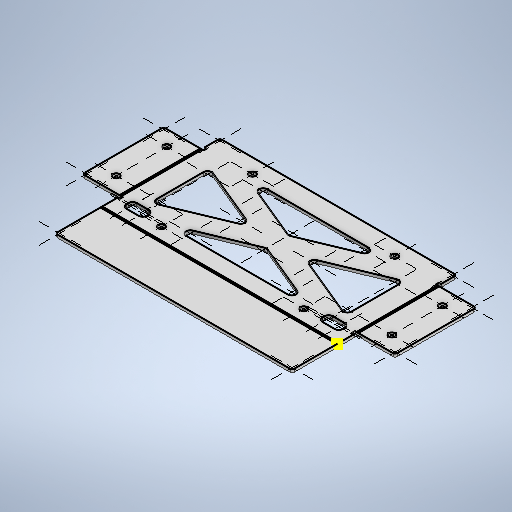
# Autodesk Inventor part: body_back_frame
Saved by Autodesk Inventor 2026.1 (Build 301233000, 233)
## iProperties
Created: 2025-08-15
Part Number: body_back_frame
Material: Generic
Document SubType Name: Modeling
Designer: chris
Density: 1 g/cm^3
Appearance: Default
Author: chris
Autodesk Inventor part; units mm, degrees
ref_plane "YZ Plane" through (0, 0, 0) normal (1, 0, 0) x (0, 1, 0)
ref_plane "XZ Plane" through (0, 0, 0) normal (0, 1, 0) x (-1, 0, 0)
ref_plane "XY Plane" through (0, 0, 0) normal (0, 0, 1) x (1, 0, 0)
sketch "Sketch1" plane through (0, 0, 0) normal (0, 1, 0) x (-1, 0, 0)
  line L0 (117, -0.4496) -> (0, -0.4496)
  line L1 (-0.1396, -9.9943) -> (-0.1396, -49.9943)
  line L2 (117.1396, -49.9943) -> (117.1396, -9.9943)
  circle A0 centre (93.69, -51.8993) radius 1.55
  circle A1 centre (23.31, -51.8993) radius 1.55
  circle A2 centre (93.69, -6.8993) radius 1.55
  circle A3 centre (23.31, -6.8993) radius 1.55
  arc A4 (15, -7.8993) -> (13, -5.8993) centre (13, -7.8993) ccw
  line L3 (7, -5.8993) -> (13, -5.8993)
  arc A5 (13, -10.8993) -> (15, -8.8993) centre (13, -8.8993) ccw
  line L4 (15, -7.8993) -> (15, -8.8993)
  arc A6 (5, -8.8993) -> (7, -10.8993) centre (7, -8.8993) ccw
  line L5 (5, -8.8993) -> (5, -7.8993)
  arc A7 (7, -5.8993) -> (5, -7.8993) centre (7, -7.8993) ccw
  arc A8 (110, -10.8993) -> (112, -8.8993) centre (110, -8.8993) ccw
  line L6 (112, -7.8993) -> (112, -8.8993)
  arc A9 (102, -8.8993) -> (104, -10.8993) centre (104, -8.8993) ccw
  line L7 (102, -8.8993) -> (102, -7.8993)
  arc A10 (112, -7.8993) -> (110, -5.8993) centre (110, -7.8993) ccw
  line L8 (104, -5.8993) -> (110, -5.8993)
  arc A11 (104, -5.8993) -> (102, -7.8993) centre (104, -7.8993) ccw
  arc A12 (13.0766, -15.651) -> (10.31, -17.4982) centre (12.31, -17.4982) ccw
  line L9 (10.31, -40.6803) -> (10.31, -17.4982)
  arc A13 (41.0052, -30.9365) -> (41.0052, -27.2421) centre (40.2386, -29.0893) ccw
  line L10 (13.0766, -15.651) -> (41.0052, -27.2421)
  arc A14 (10.31, -40.6803) -> (13.0766, -42.5275) centre (12.31, -40.6803) ccw
  line L11 (41.0052, -30.9365) -> (13.0766, -42.5275)
  arc A15 (32.6238, -45.2421) -> (33.3904, -49.0893) centre (33.3904, -47.0893) ccw
  line L12 (32.6238, -45.2421) -> (57.7334, -34.821)
  arc A16 (83.6096, -49.0893) -> (84.3762, -45.2421) centre (83.6096, -47.0893) ccw
  line L13 (59.2666, -34.821) -> (84.3762, -45.2421)
  arc A17 (59.2666, -34.821) -> (57.7334, -34.821) centre (58.5, -36.6682) ccw
  arc A18 (75.9948, -27.2421) -> (75.9948, -30.9365) centre (76.7614, -29.0893) ccw
  line L14 (75.9948, -27.2421) -> (103.9234, -15.651)
  arc A19 (106.69, -17.4982) -> (103.9234, -15.651) centre (104.69, -17.4982) ccw
  line L15 (106.69, -17.4982) -> (106.69, -40.6803)
  arc A20 (103.9234, -42.5275) -> (106.69, -40.6803) centre (104.69, -40.6803) ccw
  arc A21 (57.7334, -23.3576) -> (59.2666, -23.3576) centre (58.5, -21.5104) ccw
  line L16 (84.3762, -12.9365) -> (59.2666, -23.3576)
  arc A22 (84.3762, -12.9365) -> (83.6096, -9.0893) centre (83.6096, -11.0893) ccw
  line L17 (33.3904, -9.0893) -> (83.6096, -9.0893)
  arc A23 (33.3904, -9.0893) -> (32.6238, -12.9365) centre (33.3904, -11.0893) ccw
  line L18 (57.7334, -23.3576) -> (32.6238, -12.9365)
  line L19 (110, -10.8993) -> (104, -10.8993)
  line L20 (13, -10.8993) -> (7, -10.8993)
  circle A24 centre (-9.6843, -42.4943) radius 1.55
  circle A25 centre (126.6843, -42.4943) radius 1.55
  circle A26 centre (-9.6843, -17.4943) radius 1.55
  circle A27 centre (126.6843, -17.4943) radius 1.55
  line L21 (103.9234, -42.5275) -> (75.9948, -30.9365)
  line L22 (83.6096, -49.0893) -> (33.3904, -49.0893)
  arc A28 (134.7793, -49.9943) -> (135.7793, -48.9943) centre (134.7793, -48.9943) ccw
  line L23 (135.7793, -10.9943) -> (135.7793, -48.9943)
  arc A29 (135.7793, -10.9943) -> (134.7793, -9.9943) centre (134.7793, -10.9943) ccw
  arc A30 (117, 21.19) -> (116, 22.19) centre (116, 21.19) ccw
  line L24 (1, 22.19) -> (116, 22.19)
  arc A31 (116, -59.0893) -> (117, -58.0893) centre (116, -58.0893) ccw
  line L25 (116, -59.0893) -> (1, -59.0893)
  arc A32 (0, -58.0893) -> (1, -59.0893) centre (1, -58.0893) ccw
  line L26 (0, -58.0893) -> (0, -51.4943)
  arc A33 (-18.7793, -48.9943) -> (-17.7793, -49.9943) centre (-17.7793, -48.9943) ccw
  arc A34 (-17.7793, -9.9943) -> (-18.7793, -10.9943) centre (-17.7793, -10.9943) ccw
  line L27 (-17.7793, -9.9943) -> (1.06, -9.9943)
  arc A35 (1, 22.19) -> (0, 21.19) centre (1, 21.19) ccw
  line L28 (0, -8.4943) -> (0, 21.19)
  line L29 (134.7793, -49.9943) -> (115.94, -49.9943)
  line L30 (-18.7793, -48.9943) -> (-18.7793, -10.9943)
  line L31 (117, -51.4943) -> (115.94, -51.4943)
  line L32 (115.94, -51.4943) -> (115.94, -49.9943)
  line L33 (117, -51.4943) -> (117, -58.0893)
  line L34 (134.7793, -9.9943) -> (115.94, -9.9943)
  line L35 (115.94, -8.4943) -> (117, -8.4943)
  line L36 (115.94, -9.9943) -> (115.94, -8.4943)
  line L37 (0, -8.4943) -> (1.06, -8.4943)
  line L38 (1.06, -8.4943) -> (1.06, -9.9943)
  line L39 (1.06, -49.9943) -> (-17.7793, -49.9943)
  line L40 (1.06, -51.4943) -> (0, -51.4943)
  line L41 (1.06, -49.9943) -> (1.06, -51.4943)
  line L42 (117, 21.19) -> (117, -8.4943)
  line L43 (117.5893, -9.9943) -> (117.5893, -49.9943)
  line L44 (-0.5893, -49.9943) -> (-0.5893, -9.9943)
  line L45 (116.69, -49.9943) -> (116.69, -9.9943)
  line L46 (0.31, -9.9943) -> (0.31, -49.9943)
  line L47 (117, -0.8993) -> (0, -0.8993)
  line L48 (0, 0) -> (117, 0)
  constraints: 98 end point, 73 tangent, 56 point on circle, 36 centre point, 33 equal radius, 22 vertical, 20 parallel, 19 horizontal, 18 perpendicular, 18 point on line, 167 other
extrude "Extrusion1" add sketch "Sketch1" against normal blind 1.5
body "Solid1"
